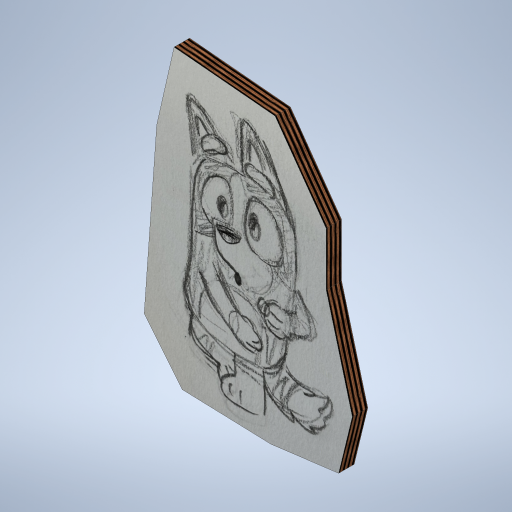
# Autodesk Inventor part: bingo
Saved by Autodesk Inventor 2023 (Build 270158000, 158)
## iProperties
Created: 2024-07-02
Part Number: bingo
Material: Generic
Document SubType Name: Modeling
Designer: Student-27
Density: 1 g/cm^3
Appearance: Default
Author: Student-27
Autodesk Inventor part; units mm, degrees
ref_plane "YZ Plane" through (0, 0, 0) normal (1, 0, 0) x (0, 1, 0)
ref_plane "XZ Plane" through (0, 0, 0) normal (0, 1, 0) x (-1, 0, 0)
ref_plane "XY Plane" through (0, 0, 0) normal (0, 0, 1) x (1, 0, 0)
sketch "Sketch1" plane through (0, 0, 0) normal (0, 0, 1) x (1, 0, 0)
  line L0 (-18.0719, 15.5659) -> (782.0281, 15.5659) construction
  line L1 (782.0281, 15.5659) -> (782.0281, -1051.2341) construction
  line L2 (782.0281, -1051.2341) -> (-18.0719, -1051.2341) construction
  line L3 (-18.0719, -1051.2341) -> (-18.0719, 15.5659) construction
  line L4 (450.0641, -291.2392) -> (533.9512, -409.0865)
  line L5 (533.9512, -409.0865) -> (533.9512, -496.2541)
  line L6 (533.9512, -496.2541) -> (556.2067, -578.785)
  line L7 (556.2067, -578.785) -> (576.8305, -655.2648)
  line L8 (576.8305, -655.2648) -> (554.4974, -746.6723)
  line L9 (554.4974, -746.6723) -> (443.3726, -760.9041)
  line L10 (443.3726, -760.9041) -> (297.7206, -756.0491)
  line L11 (297.7206, -756.0491) -> (235.4159, -678.9444)
  line L12 (235.4159, -678.9444) -> (255.9915, -400.8879)
  line L13 (255.9915, -400.8879) -> (284.4547, -276.0204)
  line L14 (284.4547, -276.0204) -> (450.0641, -291.2392)
  line L15 (576.8305, -760.9041) -> (235.4159, -760.9041)
  line L16 (235.4159, -760.9041) -> (235.4159, -276.0204)
  line L17 (235.4159, -276.0204) -> (576.8305, -276.0204)
  line L18 (576.8305, -276.0204) -> (576.8305, -760.9041)
  point P0 (0, 0)
  dimension "d7" = 341.4146
  dimension "d10" = 484.8837
  constraints: 30 end point, 2 parallel, 1 horizontal, 1 perpendicular, 1 point on line, 1 vertical, 2 other
  measures "d7" distance of L16.end L17.end
  measures "d10" distance of L17.end L15.start
extrude "Extrusion1" add sketch "Sketch1" against normal blind 25.4 contours L4 L5 L6 L7 L8 L9 L10 L11 L12 L13 L14
body "Solid1"
